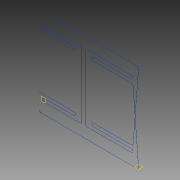
# Autodesk Inventor part: STRING GANTRY
Saved by Autodesk Inventor 2013 (Build 170138000, 138)
## iProperties
Created: 2014-06-23
Part Number: STRING GANTRY
Material: Generic
Document SubType Name: Modeling
Designer: employee
Density: 1 g/cm^3
Author: employee
Autodesk Inventor part; units mm, degrees
ref_plane "YZ Plane" through (0, 0, 0) normal (1, 0, 0) x (0, 1, 0)
ref_plane "XZ Plane" through (0, 0, 0) normal (0, 1, 0) x (-1, 0, 0)
ref_plane "Work Plane1" through (0, 0, -2.5) normal (0, 0, 1) x (1, 0, 0)
sketch "Sketch1" plane through (0, 0, -2.5) normal (0, 0, 1) x (1, 0, 0)
  circle A0 centre (-10.75, -52.5) radius 8 construction
  circle A1 centre (5.25, 0) radius 8 construction
  circle A2 centre (-10.75, 16) radius 8 construction
  circle A3 centre (248.0387, 16) radius 8 construction
  circle A4 centre (280.0387, 0) radius 8 construction
  circle A5 centre (312.0387, 0) radius 8 construction
  circle A6 centre (344.0387, 16) radius 8 construction
  circle A7 centre (452.965, -52.5) radius 9 construction
  circle A8 centre (427.965, 0) radius 8 construction
  circle A9 centre (427.965, 32) radius 8 construction
  circle A10 centre (427.965, 276) radius 8 construction
  circle A11 centre (427.965, 308) radius 8 construction
  circle A12 centre (452.965, 360.5) radius 9 construction
  circle A13 centre (344.0387, 292) radius 8 construction
  circle A14 centre (312.0387, 308) radius 8 construction
  circle A15 centre (280.0387, 308) radius 8 construction
  circle A16 centre (248.0387, 292) radius 8 construction
  circle A17 centre (-10.75, 292) radius 8 construction
  circle A18 centre (5.25, 308) radius 8 construction
  circle A19 centre (-10.75, 360.5) radius 8 construction
  line L0 (-18.75, -52.5) -> (-18.75, 16)
  line L1 (280.0387, 316) -> (5.25, 316)
  arc A20 (5.25, 316) -> (5.25, 300) centre (5.25, 308) ccw
  line L2 (5.25, 300) -> (248.0387, 300)
  line L3 (248.0387, 284) -> (-10.75, 284)
  arc A21 (248.0387, 284) -> (248.0387, 300) centre (248.0387, 292) ccw
  arc A22 (-18.75, 292) -> (-10.75, 284) centre (-10.75, 292) ccw
  line L4 (-18.75, 292) -> (-18.75, 360.5)
  line L5 (-10.7759, 368.5) -> (452.9343, 370)
  arc A23 (462.4342, 359.736) -> (452.9343, 370) centre (452.965, 360.5) ccw
  arc A24 (-10.7759, 368.5) -> (-18.75, 360.5) centre (-10.75, 360.5) ccw
  line L6 (462.4342, -51.736) -> (435.9391, 276.6434) construction
  line L7 (462.4342, 359.736) -> (435.9391, 31.3566)
  arc A25 (427.965, 24) -> (435.9391, 31.3566) centre (427.965, 32) ccw
  line L8 (427.965, 24) -> (344.0387, 24)
  arc A26 (344.0387, 24) -> (344.0387, 8) centre (344.0387, 16) ccw
  line L9 (344.0387, 8) -> (427.965, 8)
  line L10 (304.0387, 0) -> (304.0387, 308)
  line L11 (427.965, -8) -> (312.0387, -8)
  arc A27 (427.965, -8) -> (427.965, 8) centre (427.965, 0) ccw
  arc A28 (304.0387, 0) -> (312.0387, -8) centre (312.0387, 0) ccw
  line L12 (288.0387, 308) -> (288.0387, 0)
  arc A29 (288.0387, 308) -> (280.0387, 316) centre (280.0387, 308) ccw
  line L13 (280.0387, -8) -> (5.25, -8)
  line L14 (5.25, 8) -> (248.0387, 8)
  line L15 (-10.75, 24) -> (248.0387, 24)
  arc A30 (-10.75, 24) -> (-18.75, 16) centre (-10.75, 16) ccw
  arc A31 (248.0387, 8) -> (248.0387, 24) centre (248.0387, 16) ccw
  arc A32 (5.25, 8) -> (5.25, -8) centre (5.25, 0) ccw
  line L16 (312.0387, 316) -> (427.965, 316)
  arc A33 (452.9343, -62) -> (462.4342, -51.736) centre (452.965, -52.5) ccw
  line L17 (-10.7759, -60.5) -> (452.9343, -62)
  arc A34 (-18.75, -52.5) -> (-10.7759, -60.5) centre (-10.75, -52.5) ccw
  arc A35 (280.0387, -8) -> (288.0387, 0) centre (280.0387, 0) ccw
  arc A36 (312.0387, 316) -> (304.0387, 308) centre (312.0387, 308) ccw
  line L18 (427.965, 300) -> (344.0387, 300)
  line L19 (344.0387, 284) -> (427.965, 284)
  arc A37 (344.0387, 300) -> (344.0387, 284) centre (344.0387, 292) ccw
  arc A38 (435.9391, 276.6434) -> (427.965, 284) centre (427.965, 276) ccw
  arc A39 (427.965, 300) -> (427.965, 316) centre (427.965, 308) ccw
  dimension "d2" = 0.5
  dimension "d4" = 0.5
  constraints: 76 point on circle, 56 tangent, 40 end point, 20 centre point, 6 concentric, 4 coincident, 1 parallel
  measures "d2" radial gap between concentric circles of A23 A12
  measures "d4" radial gap between concentric circles of A7 A33
ref_plane "Work Plane2" through (462.4342, -51.736, -2.5) normal (-0.0804232, 0.9967608, 0) x (-0.9967608, -0.0804232, 0)
sketch "Sketch2" plane through (462.4342, -51.736, -2.5) normal (-0.0804232, 0.9967608, 0) x (-0.9967608, -0.0804232, 0)
  circle A0 centre (0, 0) radius 0.5
  point P0 (456.7755, 2.5)
  dimension "d5" = 1
  constraints: 1 centre point, 1 coincident
  measures "d5" diameter of A0
sweep "Sweep1" add profiles "Sketch2" path "Sketch1"
sketch "Sketch3" plane through (462.4342, -51.736, -2.5) normal (-0.0804232, 0.9967608, 0) x (0.9967608, 0.0804232, 0)
  circle A0 centre (0, 0) radius 0.5 projected
  point P0 (-456.7755, -2.5)
extrude "Extrusion1" add sketch "Sketch3" along normal up to surface (329.4465 mm away)
body "Solid1"
